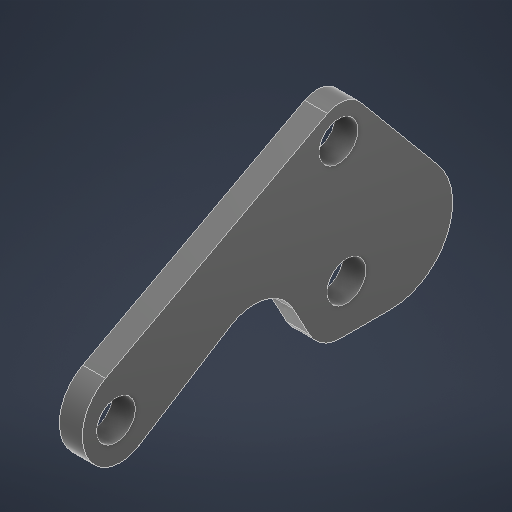
# Autodesk Inventor part: Palanca_barra
Saved by Autodesk Inventor 2027 (Build 310192060, 192F)
## iProperties
Created: 2026-06-11
Part Number: Palanca_barra
Material: Genérico
Document SubType Name: Modeling
Designer: angel
Density: 1 g/cm^3
Appearance: Suave - Negro
Author: angel
Autodesk Inventor part; units mm, degrees
ref_plane "YZ Plane" through (0, 0, 0) normal (1, 0, 0) x (0, 1, 0)
ref_plane "XZ Plane" through (0, 0, 0) normal (0, 1, 0) x (-1, 0, 0)
ref_plane "XY Plane" through (0, 0, 0) normal (0, 0, 1) x (1, 0, 0)
sketch "Boceto1" plane through (0, 0, 0) normal (1, 0, 0) x (0, 1, 0)
  line L0 (0, 0) -> (0, -65)
  line L1 (0, -65) -> (24, -65)
  line L2 (24, -65) -> (24, -45)
  line L3 (24, -45) -> (0, -65)
  line L4 (24, -45) -> (0, 0)
  line L5 (0, -65) -> (0, -60)
  dimension "d0" = 65
  dimension "d6" = 24
  dimension "d7" = 20
  dimension "d8" = 5
  constraints: 12 end point, 1 horizontal, 1 perpendicular, 1 point on line, 1 vertical
  measures "d0" distance of L0.start L0.end
  measures "d6" distance of L0.end L1.end
  measures "d7" distance of L1.end L2.end
  measures "d8" distance of L0.end L5.end
extrude "Extrusión1" add sketch "Boceto1" along normal blind 2.6 contours L4 L3 L0
fillet "Empalme1" radius 7 1 edges at (1.3, 0, -65)
fillet "Empalme2" radius 5 1 edges at (1.3, 0, 0)
fillet "Empalme3" radius 3 1 edges at (1.3, 24, -45)
sketch "Boceto2" plane through (2.6, 0, 0) normal (1, 0, 0) x (0, 0, -1)
  line L0 (0, 0) -> (49.1759, 26.2271)
  line L1 (42.8462, 22.8513) -> (17.6471, 9.4118) projected
  line L2 (0, 0) -> (69.4683, 0)
  arc A0 (50.0547, 0) -> (55.4323, 11.4813) centre (50.0547, 7) ccw projected
  line L3 (55.4323, 11.4813) -> (45, 24)
  line L4 (55.4323, 11.4813) -> (46.5627, 22.1248) projected
  line L5 (45, 24) -> (45, 0)
  circle A1 centre (45, 5.3) radius 2.2
  circle A2 centre (44.1, 19.5) radius 2.2
  line L6 (17.6471, 9.4118) -> (20.0129, 0)
  circle A3 centre (18.83, 4.7059) radius 2.2
  dimension "d14" = 4.4
  dimension "d15" = 5.3
  dimension "d18" = 4.4
  dimension "d19" = 0.9
  dimension "d20" = 19.5
  dimension "d21" = 4.4
  dimension "d22" = 26.17
  constraints: 10 end point, 4 point on line, 3 centre point, 2 collinear, 1 horizontal, 1 midpoint, 1 perpendicular
  measures "d14" diameter of A1
  measures "d15" distance from line of L2 A1.centre
  measures "d18" diameter of A2
  measures "d19" distance from line of L5 A2.centre
  measures "d20" distance from line of L2 A2.centre
  measures "d21" diameter of A3
  measures "d22" distance from line of L5 A3.centre
extrude "Extrusión2" cut sketch "Boceto2" against normal blind 10 contours A3 L6 | L6 A3 | A1 L5 | L5 A1 | A2 L5 | L5 A2
sketch "Boceto3" plane through (2.6, 0, 0) normal (1, 0, 0) x (0, 0, -1)
  arc A0 (17.6471, 9.4118) -> (20, 0) centre (20, 5) ccw projected
  line L0 (55.4323, 11.4813) -> (46.5627, 22.1248) projected
  line L1 (42.8462, 22.8513) -> (17.6471, 9.4118) projected
  line L2 (32.6471, 17.4118) -> (36.4118, 10.3529)
  line L3 (20, 0) -> (36.4118, 10.3529)
  line L4 (36.4118, 10.3529) -> (41.9333, 0)
  line L5 (20, 0) -> (50.0547, 0) projected
  line L6 (20, 0) -> (41.9333, 0)
  point P0 (0, 0)
  dimension "d24" = 90
  dimension "d25" = 8
  dimension "d26" = 17
  dimension "d27" = 11.7333
  constraints: 8 end point, 2 point on line, 1 collinear, 1 perpendicular
  measures "d24" angle of L1 L2
  measures "d25" distance of L2.start L2.end
  measures "d26" distance from line of L1.end L2
  measures "d27" distance of L2.end L4.end
extrude "Extrusión3" cut sketch "Boceto3" against normal blind 10 contours L3 L4 L5
fillet "Empalme4" radius 4 2 edges at (1.3, 0, -20) (1.3, 0, -41.9333)
fillet "Empalme de cara1" radius 5 1 edges at (1.3, 10.3529, -36.4118)
